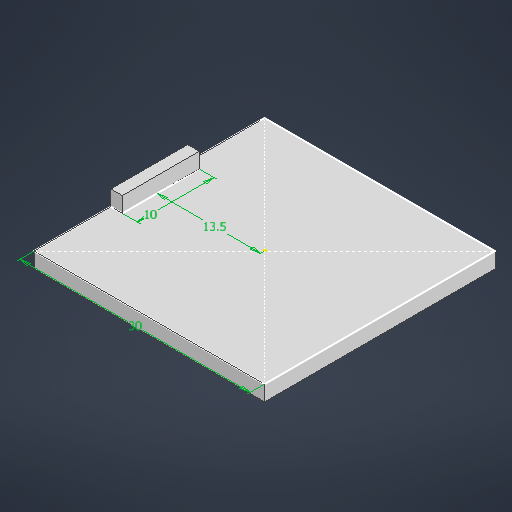
# Autodesk Inventor part: Part3
Saved by Autodesk Inventor 2025.1 (Build 291241000, 241)
## iProperties
Created: 2025-02-19
Part Number: Part3
Material: Generic
Document SubType Name: Modeling
Designer: jerem
Density: 1 g/cm^3
Appearance: Default
Author: jerem
Autodesk Inventor part; units mm, degrees
ref_plane "YZ Plane" through (0, 0, 0) normal (1, 0, 0) x (0, 1, 0)
ref_plane "XZ Plane" through (0, 0, 0) normal (0, 1, 0) x (-1, 0, 0)
ref_plane "XY Plane" through (0, 0, 0) normal (0, 0, 1) x (1, 0, 0)
sketch "Sketch1" plane through (0, 0, 0) normal (0, 1, 0) x (-1, 0, 0)
  line L0 (-15, -15) -> (15, -15)
  line L1 (15, -15) -> (15, 15)
  line L2 (15, 15) -> (-15, 15)
  line L3 (-15, 15) -> (-15, -15)
  line L4 (-15, -15) -> (15, 15) construction
  line L5 (15, -15) -> (-15, 15) construction
  line L6 (15, 5) -> (13.5, 5)
  line L7 (13.5, 5) -> (13.5, -5)
  line L8 (13.5, -5) -> (15, -5)
  line L9 (13.5, 0) -> (15, 0) construction
  point P0 (0, 0)
  dimension "d0" = 30
  dimension "d2" = 13.5
  dimension "d3" = 10
  constraints: 20 end point, 4 midpoint, 4 perpendicular, 2 horizontal, 2 parallel, 2 point on line, 1 vertical
  measures "d0" distance of L2.end L1.end
  measures "d2" distance from line of point (0, 0) L7
  measures "d3" distance of L6.end L7.end
extrude "Extrusion1" add sketch "Sketch1" against normal blind 2
extrude "Extrusion2" add sketch "Sketch1" along normal blind 2 contours L8 L7 L6 L1
body "Solid1"
